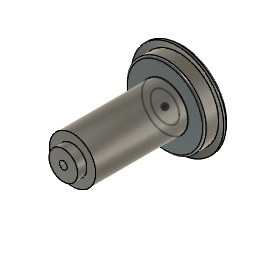
RadioGlobe-Bushing-Bottom v17 (Autodesk Fusion 360 design; units mm, degrees)
Autodesk Fusion 360 part; units mm, degrees
sketch "Sketch13" plane through (0, 0, 0) normal (0, 0, 1) x (1, 0, 0)
  line L0 (0, 105) -> (0, 100)
  arc A0 (-16.7, 100.6236) -> (-25, 98.8888) centre (0, 0) ccw
  line L1 (-25, 98.8888) -> (-25, 96.8246)
  arc A1 (-21.35, 97.6943) -> (-25, 96.8246) centre (0, 0) ccw
  line L2 (0, 90) -> (0, 100)
  line L3 (-21.35, 97.6943) -> (-21.35, 90)
  line L4 (0, 90) -> (0, 100)
  line L5 (-16.7, 100.7023) -> (-16.7, 100.6236)
  line L6 (0, 90) -> (-21.35, 90)
  line L7 (0, 105) -> (-12.5, 105)
  line L8 (-16.7, 100.7023) -> (-12.5, 100.7023)
  line L9 (-12.5, 100.7023) -> (-12.5, 105)
  dimension "d41" = 200
  dimension "d42" = 204
  dimension "d54" = 10
  dimension "d66" = 12.5
  constraint coincident A0.centre A1.centre
  constraint concentric A0 A1
  constraint vertical L0
  constraint vertical L1
  constraint vertical L2
  constraint vertical L3
  constraint vertical L4
  constraint perpendicular L3 L6
  constraint perpendicular L5 L8
  constraint perpendicular L7 L9
  measures "d41" diameter of A1
  measures "d42" diameter of A0
  measures "d54" distance of L0.end L2.start
  measures "d66" distance of L0.start L7.end
revolve "Revolve4" add sketch "Sketch13" angle 360 about axis through (0, 105, 0) along (0, -1, 0)
fillet "Fillet2" radius 1 1 edges at (-23.3082, 98.8888, 9.0404)
fillet "Fillet3" radius 1 1 edges at (-19.9052, 90, 7.7205)
sketch "Sketch16" plane through (0, 90, 0) normal (0, -1, 0) x (1, 0, 0)
  circle A0 centre (0, 0) radius 20.35
  circle A1 centre (0, 0) radius 7.75
  circle A2 centre (0, 0) radius 12.5
  dimension "d69" = 15.5
  dimension "d72" = 25
  constraint coincident A0.centre A1.centre
  constraint concentric A1 A2
  measures "d69" diameter of A1
  measures "d72" diameter of A2
extrude "Extrude7" cut sketch "Sketch16" against normal blind 30 contours A1
extrude "Extrude8" add sketch "Sketch16" along normal blind 50 contours A2
extrude "Extrude9" add sketch "Sketch16" along normal blind 55 and the other way blind -40 contours A1
sketch "Sketch18" plane through (0, 35, 0) normal (0, -1, 0) x (1, 0, 0)
  circle A0 centre (0, 0) radius 7.75
  circle A1 centre (0, 0) radius 2.1
  dimension "d80" = 4.2
  constraint coincident A0.centre A1.centre
  measures "d80" diameter of A1
extrude "Extrude10" cut sketch "Sketch18" against normal blind 86 contours A1
